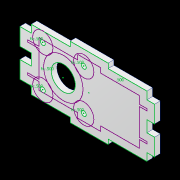
# Autodesk Inventor part: DriveSideFrame_02
Saved by Autodesk Inventor 2021 (Build 250183000, 183)
## iProperties
Created: 2021-03-08
Part Number: DriveSideFrame_02
Material: Aluminum 6061
Document SubType Name: Modeling
Designer: M3rob
Density: 2.7 g/cm^3
Appearance: Aluminum - Flat
Mass: 539.031 g
Surface Area: 512.257 cm^2
Volume: 199.641 cm^3
Author: M3rob
Autodesk Inventor part; units mm, degrees
ref_plane "YZ Plane" through (0, 0, 0) normal (1, 0, 0) x (0, 1, 0)
ref_plane "XZ Plane" through (0, 0, 0) normal (0, 1, 0) x (-1, 0, 0)
ref_plane "XY Plane" through (0, 0, 0) normal (0, 0, 1) x (1, 0, 0)
sketch "Sketch1" plane through (0, 0, 0) normal (0, 0, 1) x (1, 0, 0)
  line L0 (-96.52, 50.8) -> (-96.52, 38.1)
  line L1 (-96.52, -50.8) -> (-31.75, -50.8)
  line L2 (96.52, -50.8) -> (96.52, -38.1)
  line L3 (96.52, 50.8) -> (31.75, 50.8)
  line L4 (-96.52, 0) -> (96.52, 0) construction
  line L5 (96.52, 38.1) -> (109.22, 38.1)
  line L6 (109.22, 38.1) -> (109.22, 9.525)
  line L7 (109.22, 9.525) -> (96.52, 9.525)
  line L8 (96.52, -9.525) -> (109.22, -9.525)
  line L9 (109.22, -9.525) -> (109.22, -38.1)
  line L10 (109.22, -38.1) -> (96.52, -38.1)
  line L11 (96.52, 38.1) -> (96.52, 50.8)
  line L12 (96.52, 9.525) -> (96.52, 38.1) construction
  line L13 (96.52, -9.525) -> (96.52, 9.525)
  line L14 (96.52, -38.1) -> (96.52, -9.525) construction
  line L15 (-96.52, 6.7437) -> (-86.995, 6.7437) construction
  line L16 (-86.995, 6.7437) -> (-86.995, 9.525) construction
  line L17 (-86.995, 9.525) -> (-79.0575, 9.525) construction
  line L18 (-79.0575, 9.525) -> (-79.0575, 6.7437) construction
  line L19 (-79.0575, 6.7437) -> (-75.8825, 6.7437) construction
  line L20 (-75.8825, 6.7437) -> (-75.8825, -6.7437) construction
  line L21 (-75.8825, -6.7437) -> (-79.0575, -6.7437) construction
  line L22 (-79.0575, -6.7437) -> (-79.0575, -9.525) construction
  line L23 (-79.0575, -9.525) -> (-86.995, -9.525) construction
  line L24 (-86.995, -9.525) -> (-86.995, -6.7437) construction
  line L25 (-86.995, -6.7437) -> (-96.52, -6.7437) construction
  line L26 (-96.52, 6.7437) -> (-96.52, -6.7437)
  line L27 (-96.52, -6.7437) -> (-96.52, -9.525)
  line L28 (-31.75, 50.8) -> (-31.75, 58.7375)
  line L29 (-31.75, 58.7375) -> (31.75, 58.7375)
  line L30 (31.75, 58.7375) -> (31.75, 50.8)
  line L31 (-31.75, -50.8) -> (-31.75, -58.7375)
  line L32 (-31.75, -58.7375) -> (31.75, -58.7375)
  line L33 (31.75, -58.7375) -> (31.75, -50.8)
  line L34 (-31.75, 50.8) -> (-96.52, 50.8)
  line L35 (31.75, 50.8) -> (-31.75, 50.8) construction
  line L36 (31.75, -50.8) -> (96.52, -50.8)
  line L37 (-31.75, -50.8) -> (31.75, -50.8) construction
  line L38 (-96.52, 38.1) -> (-115.57, 38.1)
  line L39 (-115.57, 38.1) -> (-115.57, 9.525)
  line L40 (-115.57, 9.525) -> (-96.52, 9.525)
  line L41 (-96.52, -9.525) -> (-115.57, -9.525)
  line L42 (-115.57, -9.525) -> (-115.57, -38.1)
  line L43 (-115.57, -38.1) -> (-96.52, -38.1)
  line L44 (-96.52, 38.1) -> (-96.52, 9.525) construction
  line L45 (-96.52, 9.525) -> (-96.52, 6.7437)
  line L46 (-96.52, -9.525) -> (-96.52, -38.1) construction
  line L47 (-96.52, -38.1) -> (-96.52, -50.8)
  circle A0 centre (-43.18, 0) radius 7.9375
  circle A1 centre (-43.18, 0) radius 20.066
  point P0 (0, 0)
  point P1 (0, 0)
  point P2 (0, 58.7375)
  point P3 (0, -58.7375)
  point P4 (109.22, 23.8125)
  point P5 (-96.52, 6.35)
  point P6 (-96.52, -6.35)
  dimension "d0" = 101.6
  dimension "d1" = 193.04
  dimension "d2" = 19.05
  dimension "d3" = 12.7
  dimension "d4" = 12.7
  dimension "d5" = 13.4874
  dimension "d6" = 9.525
  dimension "d7" = 7.9375
  dimension "d8" = 3.175
  dimension "d9" = 19.05
  dimension "d10" = 63.5
  dimension "d11" = 7.9375
  dimension "d12" = 19.05
  dimension "d13" = 53.34
  dimension "d14" = 15.875
  dimension "d17" = 40.132
  constraints: 96 end point, 66 perpendicular, 39 parallel, 11 point on line, 9 vertical, 6 midpoint, 3 equal length, 3 horizontal, 3 symmetric about line, 2 centre point, 2 coincident, 2 horizontal alignment, 2 vertical alignment, 7 other
  measures "d0" distance of L0.start L1.start
  measures "d1" distance of L3.start L0.start
  measures "d2" diameter of L7 L4
  measures "d3" distance of L3.start L5.start
  measures "d4" distance of L5.start L5.end
  measures "d5" distance between parallel lines of L25 L15
  measures "d6" distance of L15.start L15.end
  measures "d7" distance of L16.end L17.end
  measures "d8" distance of L18.end L19.end
  measures "d9" distance between parallel lines of L23 L17
  measures "d10" distance of L28.end L29.end
  measures "d11" distance of L32.end L33.end
  measures "d12" distance of L0.end L38.end
  measures "d13" horizontal distance of L27.end A0.centre
  measures "d14" diameter of A0
  measures "d17" diameter of A1
extrude "Extrusion2" add sketch "Sketch1" along normal blind 9.525 contours L34 L28 L29 L30 L3 L11 L5 L6 L7 L13 L8 L9 L10 L2 L36 L33 L32 L31 L1 L47 L43 L42 L41 L27 L26 L45 L40 L39 L38 L0
sketch "Sketch2" plane through (0, 0, 9.525) normal (0, 0, 1) x (1, 0, 0)
  circle A0 centre (-43.18, 0) radius 27.8049
  circle A1 centre (-43.18, 0) radius 20.066 projected
  line L0 (-77.343, -34.163) -> (-9.017, -34.163) construction
  line L1 (-9.017, -34.163) -> (-77.343, -34.163) construction
  line L2 (-77.343, -34.163) -> (-77.343, 34.163) construction
  line L3 (-77.343, 34.163) -> (-9.017, 34.163) construction
  line L4 (-9.017, 34.163) -> (-9.017, -34.163) construction
  line L5 (-9.017, -34.163) -> (-77.343, 34.163) construction
  line L6 (-77.343, -34.163) -> (-9.017, 34.163) construction
  point P0 (-9.017, 34.163)
  point P1 (-43.18, 27.9401)
  point P2 (-84.4499, 0)
  dimension "d34" = 68.326
  dimension "d35" = 68.326
  constraints: 14 end point, 2 horizontal, 2 midpoint, 2 parallel, 1 centre point, 1 coincident, 1 concentric, 1 horizontal alignment, 1 perpendicular, 1 vertical alignment
  measures "d34" distance of L2.end L3.end
  measures "d35" distance of L0.start L2.end
hole "Hole1" at (-77.343, 34.163, 9.525) at (-9.017, 34.163, 9.525) at (-77.343, -34.163, 9.525) at (-9.017, -34.163, 9.525) direction (0, 0, -1) diameter 8.1915 end through all
sketch "Sketch3" plane through (0, 0, 9.525) normal (0, 0, 1) x (1, 0, 0)
  line L0 (96.52, 50.8) -> (31.75, 50.8) projected
  line L1 (96.52, 38.1) -> (96.52, 50.8) projected
  line L2 (31.75, -50.8) -> (96.52, -50.8) projected
  line L3 (96.52, -50.8) -> (96.52, -38.1) projected
  circle A0 centre (-9.017, 34.163) radius 4.0957 projected
  circle A1 centre (-9.017, -34.163) radius 4.0957 projected
  line L4 (96.52, 50.8) -> (83.82, 50.8)
  line L5 (83.82, 50.8) -> (83.82, 38.1) construction
  line L6 (83.82, 38.1) -> (96.52, 38.1) construction
  line L7 (96.52, 38.1) -> (96.52, 50.8)
  line L8 (96.52, -50.8) -> (83.82, -50.8)
  line L9 (83.82, -50.8) -> (83.82, -38.1) construction
  line L10 (83.82, -38.1) -> (96.52, -38.1) construction
  line L11 (96.52, -38.1) -> (96.52, -50.8)
  line L12 (-4.9212, 34.163) -> (7.7788, 34.163) construction
  line L13 (-31.75, -58.7375) -> (31.75, -58.7375) projected
  line L14 (83.82, -38.1) -> (83.82, 38.1)
  line L15 (83.82, 38.1) -> (-10.414, 0) construction
  line L16 (83.82, -38.1) -> (-10.414, 0) construction
  circle A2 centre (-43.18, 0) radius 20.066 projected
  line L17 (-23.114, 0) -> (-10.414, 0) construction
  line L18 (83.82, 0) -> (83.82, 6.35)
  line L19 (83.82, 0) -> (83.82, -6.35)
  line L20 (83.82, 6.35) -> (162.3483, 6.35) construction
  line L21 (83.82, -6.35) -> (5.2917, -6.35)
  line L22 (31.75, 50.8) -> (83.82, 50.8)
  line L23 (83.82, 50.8) -> (83.82, 38.1)
  line L24 (83.82, 38.1) -> (31.75, 38.1) construction
  line L25 (31.75, 38.1) -> (31.75, 50.8) construction
  line L26 (-10.414, 6.35) -> (-10.414, -6.35)
  line L27 (-10.414, -6.35) -> (5.2917, -6.35)
  line L28 (83.82, 6.35) -> (-10.414, 6.35)
  line L29 (36.703, 6.35) -> (36.703, 38.1) construction
  line L30 (36.703, 6.35) -> (36.703, -50.8) construction
  line L31 (31.75, -50.8) -> (96.52, -50.8) construction
  line L32 (-10.414, 6.35) -> (36.703, 38.1)
  line L33 (83.82, 6.35) -> (36.703, 38.1)
  line L34 (36.703, -50.8) -> (36.703, -38.1) construction
  line L35 (-10.414, -6.35) -> (36.703, -38.1)
  line L36 (83.82, -6.35) -> (36.703, -38.1)
  circle A3 centre (-9.017, 34.163) radius 16.7958 construction
  line L37 (36.703, 6.35) -> (43.053, 6.35)
  line L38 (36.703, 6.35) -> (30.353, 6.35)
  line L39 (43.053, 6.35) -> (43.053, 33.821)
  line L40 (30.353, 6.35) -> (30.353, 33.821)
  line L41 (43.053, 6.35) -> (43.053, -6.35) construction
  line L42 (30.353, 6.35) -> (30.353, -6.35) construction
  line L43 (43.053, -6.35) -> (43.053, -33.821)
  line L44 (30.353, -6.35) -> (30.353, -33.821)
  point P0 (0, 0)
  dimension "d36" = 12.7
  dimension "d37" = 12.7
  dimension "d38" = 12.7
  dimension "d39" = 12.7
  dimension "d40" = 12.7
  dimension "d42" = 12.7
  dimension "d46" = 6.35
  dimension "d47" = 6.35
  dimension "d49" = 12.7
  dimension "d50" = 6.35
  dimension "d51" = 6.35
  constraints: 78 end point, 15 point on line, 9 perpendicular, 8 parallel, 7 horizontal, 3 horizontal alignment, 2 midpoint, 2 vertical, 1 coincident, 4 other
  measures "d36" distance of L6.end L5.end
  measures "d37" distance of L5.end L4.end
  measures "d38" distance of L9.end L10.end
  measures "d39" distance of L8.end L9.end
  measures "d40" distance of L12.start L12.end
  measures "d42" distance of L17.start L15.end
  measures "d46" distance of L18.start L18.end
  measures "d47" distance of L18.start L19.end
  measures "d49" distance of L30.end L34.end
  measures "d50" distance of L29.start L37.end
  measures "d51" distance of L29.start L38.end
extrude "Extrusion3" [suppressed]
fillet "Fillet1" [suppressed]
sketch "Sketch4" plane through (0, 0, 9.525) normal (0, 0, 1) x (1, 0, 0)
  circle A0 centre (-77.343, -34.163) radius 4.0957 projected
  circle A1 centre (-77.343, 34.163) radius 4.0957 projected
  circle A2 centre (-9.017, 34.163) radius 4.0957 projected
  circle A3 centre (-9.017, -34.163) radius 4.0957 projected
  line L0 (-96.52, 50.8) -> (-96.52, 38.1) projected
  line L1 (-96.52, 38.1) -> (-115.57, 38.1) projected
  line L2 (-115.57, 38.1) -> (-115.57, 9.525) projected
  line L3 (-115.57, 9.525) -> (-96.52, 9.525) projected
  line L4 (-96.52, 9.525) -> (-96.52, -9.525) projected
  line L5 (-96.52, -9.525) -> (-115.57, -9.525) projected
  line L6 (-115.57, -9.525) -> (-115.57, -38.1) projected
  line L7 (-115.57, -38.1) -> (-96.52, -38.1) projected
  line L8 (-96.52, -38.1) -> (-96.52, -50.8) projected
  line L9 (-96.52, -50.8) -> (-31.75, -50.8) projected
  line L10 (-31.75, -50.8) -> (-31.75, -58.7375) projected
  line L11 (-31.75, -58.7375) -> (31.75, -58.7375) projected
  line L12 (31.75, -58.7375) -> (31.75, -50.8) projected
  line L13 (31.75, -50.8) -> (96.52, -50.8) projected
  line L14 (96.52, -50.8) -> (96.52, -38.1) projected
  line L15 (96.52, -38.1) -> (109.22, -38.1) projected
  line L16 (109.22, -38.1) -> (109.22, -9.525) projected
  line L17 (109.22, -9.525) -> (96.52, -9.525) projected
  line L18 (96.52, -9.525) -> (96.52, 9.525) projected
  line L19 (96.52, 9.525) -> (109.22, 9.525) projected
  line L20 (109.22, 9.525) -> (109.22, 38.1) projected
  line L21 (109.22, 38.1) -> (96.52, 38.1) projected
  line L22 (96.52, 38.1) -> (96.52, 50.8) projected
  line L23 (96.52, 50.8) -> (31.75, 50.8) projected
  line L24 (31.75, 50.8) -> (31.75, 58.7375) projected
  line L25 (31.75, 58.7375) -> (-31.75, 58.7375) projected
  line L26 (-31.75, 58.7375) -> (-31.75, 50.8) projected
  line L27 (-31.75, 50.8) -> (-96.52, 50.8) projected
  circle A4 centre (-43.18, 0) radius 20.066 projected
  line L28 (19.05, 38.1) -> (83.82, 38.1)
  line L29 (83.82, 38.1) -> (83.82, 25.4)
  line L30 (83.82, 25.4) -> (96.52, 25.4)
  line L31 (96.52, 25.4) -> (96.52, 22.225)
  line L32 (96.52, 22.225) -> (83.82, 22.225)
  line L33 (83.82, 22.225) -> (83.82, -22.225)
  line L34 (83.82, -22.225) -> (96.52, -22.225)
  line L35 (96.52, -22.225) -> (96.52, -25.4)
  line L36 (96.52, -25.4) -> (83.82, -25.4)
  line L37 (83.82, -25.4) -> (83.82, -38.1)
  line L38 (83.82, -38.1) -> (19.05, -38.1)
  line L39 (19.05, -38.1) -> (19.05, -46.0375)
  line L40 (19.05, -46.0375) -> (-19.05, -46.0375)
  line L41 (-19.05, -46.0375) -> (-19.05, -38.1)
  line L42 (-19.05, -38.1) -> (-83.82, -38.1)
  line L43 (-83.82, -38.1) -> (-83.82, -25.4)
  line L44 (-83.82, -25.4) -> (-102.87, -25.4)
  line L45 (-102.87, -25.4) -> (-102.87, -22.225)
  line L46 (-102.87, -22.225) -> (-83.82, -22.225)
  line L47 (-83.82, -22.225) -> (-83.82, 22.225)
  line L48 (-83.82, 22.225) -> (-102.87, 22.225)
  line L49 (-102.87, 22.225) -> (-102.87, 25.4)
  line L50 (-102.87, 25.4) -> (-83.82, 25.4)
  line L51 (-83.82, 25.4) -> (-83.82, 38.1)
  line L52 (-83.82, 38.1) -> (-19.05, 38.1)
  line L53 (-19.05, 38.1) -> (-19.05, 46.0375)
  line L54 (-19.05, 46.0375) -> (19.05, 46.0375)
  line L55 (19.05, 46.0375) -> (19.05, 38.1)
  circle A5 centre (-9.017, 34.163) radius 16.7958
  circle A6 centre (-77.343, 34.163) radius 16.7958
  circle A7 centre (-9.017, -34.163) radius 16.7958
  circle A8 centre (-77.343, -34.163) radius 16.7958
  circle A9 centre (-43.18, 0) radius 32.766
  point P0 (0, 0)
  dimension "t" = 12.7
  dimension "d53" = 12.7
  dimension "d54" = 12.7
  dimension "d55" = 12.7
  dimension "d56" = 12.7
  dimension "d57" = 12.7
  constraints: 56 end point, 5 centre point, 27 other
  measures "t" distance between parallel lines of L23 L28
  measures "d53" radial gap between concentric circles of A2 A5
  measures "d54" radial gap between concentric circles of A1 A6
  measures "d55" radial gap between concentric circles of A3 A7
  measures "d56" radial gap between concentric circles of A0 A8
  measures "d57" radial gap between concentric circles of A4 A9
equation "\"d53\" = t"
equation "\"d54\" = t"
equation "\"d55\" = t"
equation "\"d56\" = t"
equation "\"d57\" = t"
body "Solid2"
